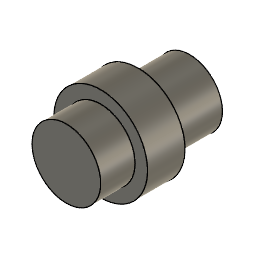
Untitled (Autodesk Fusion 360 design; units mm, degrees)
Autodesk Fusion 360 part; units mm, degrees
sketch "Sketch1" plane through (0, 0, 0) normal (0, 1, 0) x (1, 0, 0)
  circle A0 centre (-40, -20) radius 1.5
  dimension "d1" = 3
  measures "d1" diameter of A0
extrude "Extrude1" add sketch "Sketch1" along normal blind 1.2
sketch "Sketch2" plane through (0, 0, 0) normal (0, -1, 0) x (1, 0, 0)
  circle A0 centre (-40, 20) radius 1.5
  circle A1 centre (-40, 20) radius 1.1
  dimension "d4" = 2.2
  constraint concentric A0 A1
  measures "d4" diameter of A1
extrude "Extrude2" add sketch "Sketch2" along normal blind 1.1 contours A1
sketch "Sketch3" plane through (0, 1.2, 0) normal (0, 1, 0) x (-1, 0, 0)
  circle A0 centre (40, 20) radius 1.5
  circle A1 centre (40, 20) radius 1.05
  dimension "d7" = 2.1
  constraint concentric A0 A1
  measures "d7" diameter of A1
extrude "Extrude3" add sketch "Sketch3" along normal blind 1.65 contours A1
